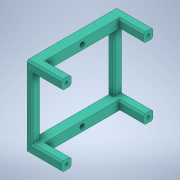
# Autodesk Inventor part: batt-standoff
Saved by Autodesk Inventor 2020 (Build 240168000, 168)
## iProperties
Created: 2020-11-07
Part Number: batt-standoff
Material: Generic
Document SubType Name: Modeling
Designer: alnwlsn
Density: 1 g/cm^3
Appearance: Default
Author: alnwlsn
Autodesk Inventor part; units mm, degrees
ref_plane "YZ Plane" through (0, 0, 0) normal (1, 0, 0) x (0, 1, 0)
ref_plane "XZ Plane" through (0, 0, 0) normal (0, 1, 0) x (-1, 0, 0)
ref_plane "XY Plane" through (0, 0, 0) normal (0, 0, 1) x (1, 0, 0)
sketch "Sketch1" plane through (0, 0, 0) normal (0, 1, 0) x (-1, 0, 0)
  line L0 (0, 0) -> (22, 0)
  line L1 (22, 0) -> (22, -58)
  line L2 (22, -58) -> (0, -58)
  line L3 (0, -58) -> (0, -52)
  line L4 (0, -52) -> (16, -52)
  line L5 (16, -52) -> (16, -6)
  line L6 (16, -6) -> (0, -6)
  line L7 (0, -6) -> (0, 0)
  dimension "d0" = 6
  dimension "d1" = 6
  dimension "d2" = 58
  dimension "d3" = 22
  constraints: 16 end point, 7 perpendicular, 1 collinear, 1 horizontal, 1 point on line
  measures "d0" distance between parallel lines of L5 L1
  measures "d1" distance between parallel lines of L6 L0
  measures "d2" distance between parallel lines of L2 L0
  measures "d3" distance of L0.start L0.end
extrude "Extrusion1" add sketch "Sketch1" along normal blind 6
sketch "Sketch2" plane through (0, 0, 0) normal (1, 0, 0) x (0, 0, -1)
  line L0 (6, 6) -> (52, 6) projected
  line L1 (0, 0) -> (6, 6) construction
  line L2 (58, 0) -> (58, 6) projected
  line L3 (52, 6) -> (58, 0) construction
  circle A0 centre (3, 3) radius 1
  circle A1 centre (55, 3) radius 1
  dimension "d6" = 2
  constraints: 4 end point, 2 centre point, 2 midpoint, 1 equal radius, 1 perpendicular
  measures "d6" diameter of A1
extrude "Extrusion2" cut sketch "Sketch2" against normal blind 12
sketch "Sketch3" plane through (-16, 0, -6) normal (1, 0, 0) x (0, 0, -1)
  line L0 (0, 6) -> (46, 6) projected
  line L1 (23, 6) -> (23, 0) construction
  circle A0 centre (23, 3) radius 1.5
  line L2 (0, 0) -> (46, 0) projected
  point P0 (-6, 0)
  dimension "d9" = 3
  constraints: 3 midpoint, 2 end point, 1 centre point, 1 vertical
  measures "d9" diameter of A0
extrude "Extrusion3" cut sketch "Sketch3" against normal through all
pattern_linear "Rectangular Pattern2" count 2 spacing 45 along (0, 1, 0) of "Extrusion1", "Extrusion3", "Extrusion2"
sketch "Sketch5" plane through (-22, 0, -58) normal (-1, 0, 0) x (0, 0, 1)
  line L0 (58, 0) -> (52, 0) projected
  line L1 (52, 51) -> (6, 51) projected
  line L2 (58, 0) -> (52, 0)
  line L3 (52, 0) -> (52, 51)
  line L4 (52, 51) -> (58, 51)
  line L5 (58, 51) -> (58, 0)
  line L6 (6, 0) -> (0, 0) projected
  line L7 (6, 45) -> (6, 51) projected
  line L8 (0, 0) -> (6, 0)
  line L9 (6, 0) -> (6, 51)
  line L10 (6, 51) -> (0, 51)
  line L11 (0, 51) -> (0, 0)
  constraints: 16 end point, 4 parallel, 2 horizontal, 2 perpendicular
extrude "Extrusion4" add sketch "Sketch5" against normal blind 3
chamfer "Chamfer3" distance 1 angle 45 20 edges at (-11, 51, 0) (-9.5, 45, 0) (-8, 51, -6) (-8, 45, -52) (-8, 51, -52) (-11, 51, -58) (-9.5, 6, -58) (-8, 6, -52) (-8, 0, -52) (-8, 6, -6) (-9.5, 6, 0) (-11, 0, 0) (-8, 45, -6) (-8, 0, -6) (-11, 0, -58) (-9.5, 45, -58) (-19, 25.5, -6) (-19, 25.5, 0) (-19, 25.5, -52) (-19, 25.5, -58)
body "Solid1"
